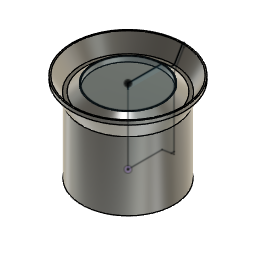
stackable-container (Autodesk Fusion 360 design; units mm, degrees)
Autodesk Fusion 360 part; units mm, degrees
note: some values were not read from the file. Set by a fixed rule: which sketch regions a step uses.
sketch "Sketch1" plane through (0, 0, 0) normal (1, 0, 0) x (0, 1, 0)
  line L0 (0, 0) -> (10.4, 0)
  line L1 (13.2, -2.3495) -> (14, -2.3495)
  line L2 (14, -2.3495) -> (14, 18.4689)
  line L3 (13.1, 20.4689) -> (10.5, 22.6505)
  line L4 (10.5, 22.6505) -> (0, 22.6505)
  line L5 (0, 22.6505) -> (0, 0)
  line L6 (14, -2.3495) -> (14, -3.0208) construction
  line L7 (10.4, 0) -> (14, -3.0208)
  line L8 (16.6, 24.799) -> (14.1, 20.4689)
  line L9 (14.1, 20.4689) -> (13.1, 20.4689)
  line L10 (14, 18.4689) -> (17, 23.665)
  line L11 (16.6, 24.799) -> (17, 24.799)
  line L12 (17, 24.799) -> (17, 23.665)
  dimension "d1" = 14
  dimension "d2" = 25
  dimension "d4" = 0.8
  dimension "d10" = 140
  dimension "d11" = 10.4
  dimension "d12" = 10.5
  dimension "d13" = 2.3495
  dimension "d14" = 1
  dimension "d15" = 0.1
  dimension "d16" = 60
  dimension "d17" = 150
  dimension "d18" = 2.1817
  dimension "d19" = 2
  dimension "d20" = 0.4
  dimension "d21" = 17
  constraint coincident L0.start L5.end
  constraint horizontal L0
  constraint parallel L0 L1
  constraint perpendicular L1 L2
  constraint perpendicular L2 L4
  constraint perpendicular L0 L5
  constraint perpendicular L1 L6
  constraint coincident L1.start L7
  constraint parallel L3 L7
  constraint perpendicular L2 L9
  constraint coincident L2 L10.start
  constraint perpendicular L11 L12
  constraint coincident L10.end L12.end
  constraint horizontal L11
  measures "d1" distance of L2 L5
  measures "d2" distance of L1 L4
  measures "d4" distance of L1.start L1.end
  measures "d10" angle of L0 L7
  measures "d11" distance of L0.end L5
  measures "d12" distance of L3.end L4.end
  measures "d13" distance of L0 L1
  measures "d14" distance of L3.start L8.end
  measures "d15" distance of L2 L8.end
  measures "d16" angle of L8 L9
  measures "d17" angle of L2 L10
  measures "d18" distance of L4 L9
  measures "d19" vertical distance of L8.end L2.end
  measures "d20" distance of L8.start L11.end
  measures "d21" distance of L5 L12
revolve "Revolve1" add sketch "Sketch1" angle 360 about axis through (0, 0, 22.6505) along (0, 0, -1)
sketch "Sketch2" plane through (0, 0, 22.6505) normal (0, 0, 1) x (-1, 0, 0)
  circle A0 centre (0, 0) radius 10.5
  circle A1 centre (0, 0) radius 10.25
  dimension "d7" = 20.5
  constraint concentric A0 A1
  measures "d7" diameter of A1
extrude "Extrude1" cut sketch "Sketch2" against normal blind 1.6 contours A1
equation "d1 = ( 28 / 2 ) * 1 mm"
